Autodesk Inventor part; units mm, degrees
(part 3 of 3)
  line L455 (50.25, -72.75) -> (50.25, -62.25)
  line L456 (50.25, -62.25) -> (24.75, -62.25)
  line L457 (24.75, -62.25) -> (24.75, -72.75)
  line L458 (24.75, -57.75) -> (50.25, -57.75)
  line L459 (50.25, -57.75) -> (50.25, -47.25)
  line L460 (50.25, -47.25) -> (24.75, -47.25)
  line L461 (24.75, -47.25) -> (24.75, -57.75)
  line L462 (24.75, -42.75) -> (50.25, -42.75)
  line L463 (50.25, -42.75) -> (50.25, -32.25)
  line L464 (50.25, -32.25) -> (24.75, -32.25)
  line L465 (24.75, -32.25) -> (24.75, -42.75)
  line L466 (24.75, -27.75) -> (50.25, -27.75)
  line L467 (50.25, -27.75) -> (50.25, -17.25)
  line L468 (50.25, -17.25) -> (24.75, -17.25)
  line L469 (24.75, -17.25) -> (24.75, -27.75)
  line L470 (24.75, -12.75) -> (50.25, -12.75)
  line L471 (50.25, -12.75) -> (50.25, -2.25)
  line L472 (50.25, -2.25) -> (24.75, -2.25)
  line L473 (24.75, -2.25) -> (24.75, -12.75)
  line L474 (24.75, 2.25) -> (50.25, 2.25)
  line L475 (50.25, 2.25) -> (50.25, 12.75)
  line L476 (50.25, 12.75) -> (24.75, 12.75)
  line L477 (24.75, 12.75) -> (24.75, 2.25)
  line L478 (24.75, 17.25) -> (50.25, 17.25)
  line L479 (50.25, 17.25) -> (50.25, 27.75)
  line L480 (50.25, 27.75) -> (24.75, 27.75)
  line L481 (24.75, 27.75) -> (24.75, 17.25)
  line L482 (24.75, 32.25) -> (50.25, 32.25)
  line L483 (50.25, 32.25) -> (50.25, 42.75)
  line L484 (50.25, 42.75) -> (24.75, 42.75)
  line L485 (24.75, 42.75) -> (24.75, 32.25)
  line L486 (24.75, 47.25) -> (50.25, 47.25)
  line L487 (50.25, 47.25) -> (50.25, 57.75)
  line L488 (50.25, 57.75) -> (24.75, 57.75)
  line L489 (24.75, 57.75) -> (24.75, 47.25)
  line L490 (24.75, 62.25) -> (50.25, 62.25)
  line L491 (50.25, 62.25) -> (50.25, 72.75)
  line L492 (50.25, 72.75) -> (24.75, 72.75)
  line L493 (24.75, 72.75) -> (24.75, 62.25)
  line L494 (24.75, 77.25) -> (50.25, 77.25)
  line L495 (50.25, 77.25) -> (50.25, 87.75)
  line L496 (50.25, 87.75) -> (24.75, 87.75)
  line L497 (24.75, 87.75) -> (24.75, 77.25)
  line L498 (24.75, 92.25) -> (50.25, 92.25)
  line L499 (50.25, 92.25) -> (50.25, 102.75)
  line L500 (50.25, 102.75) -> (24.75, 102.75)
  line L501 (24.75, 102.75) -> (24.75, 92.25)
  line L502 (24.75, 107.25) -> (50.25, 107.25)
  line L503 (50.25, 107.25) -> (50.25, 117.75)
  line L504 (50.25, 117.75) -> (24.75, 117.75)
  line L505 (24.75, 117.75) -> (24.75, 107.25)
  line L506 (9.75, -87.75) -> (20.25, -87.75)
  line L507 (20.25, -87.75) -> (20.25, -69.75)
  line L508 (20.25, -69.75) -> (9.75, -69.75)
  line L509 (9.75, -69.75) -> (9.75, -87.75)
  line L510 (9.75, -47.25) -> (20.25, -47.25)
  line L511 (20.25, -47.25) -> (20.25, -65.25)
  line L512 (20.25, -65.25) -> (9.75, -65.25)
  line L513 (9.75, -65.25) -> (9.75, -47.25)
  line L514 (9.75, -42.75) -> (20.25, -42.75)
  line L515 (20.25, -42.75) -> (20.25, -24.75)
  line L516 (20.25, -24.75) -> (9.75, -24.75)
  line L517 (9.75, -24.75) -> (9.75, -42.75)
  line L518 (9.75, -20.25) -> (20.25, -20.25)
  line L519 (20.25, -20.25) -> (20.25, -9.75)
  line L520 (20.25, -9.75) -> (9.75, -9.75)
  line L521 (9.75, -9.75) -> (9.75, -20.25)
  line L522 (9.75, 12.75) -> (20.25, 12.75)
  line L523 (20.25, 12.75) -> (20.25, -5.25)
  line L524 (20.25, -5.25) -> (9.75, -5.25)
  line L525 (9.75, -5.25) -> (9.75, 12.75)
  line L526 (9.75, 17.25) -> (20.25, 17.25)
  line L527 (20.25, 17.25) -> (20.25, 35.25)
  line L528 (20.25, 35.25) -> (9.75, 35.25)
  line L529 (9.75, 35.25) -> (9.75, 17.25)
  line L530 (9.75, 57.75) -> (20.25, 57.75)
  line L531 (20.25, 57.75) -> (20.25, 39.75)
  line L532 (20.25, 39.75) -> (9.75, 39.75)
  line L533 (9.75, 39.75) -> (9.75, 57.75)
  line L534 (9.75, 62.25) -> (20.25, 62.25)
  line L535 (20.25, 62.25) -> (20.25, 80.25)
  line L536 (20.25, 80.25) -> (9.75, 80.25)
  line L537 (9.75, 80.25) -> (9.75, 62.25)
  line L538 (9.75, 117.75) -> (20.25, 117.75)
  line L539 (20.25, 117.75) -> (20.25, 99.75)
  line L540 (20.25, 99.75) -> (9.75, 99.75)
  line L541 (9.75, 99.75) -> (9.75, 117.75)
  line L542 (9.75, 84.75) -> (20.25, 84.75)
  line L543 (20.25, 84.75) -> (20.25, 95.25)
  line L544 (20.25, 95.25) -> (9.75, 95.25)
  line L545 (9.75, 95.25) -> (9.75, 84.75)
  point P0 (0, 0)
  point P1 (9.75, -64.25)
  point P2 (20.25, -53.75)
  point P3 (20.25, -49.25)
  point P4 (20.25, -8.75)
  point P5 (20.25, -4.25)
  point P6 (20.25, 36.25)
  point P7 (9.75, 40.75)
  point P8 (20.25, 51.25)
  point P9 (20.25, 55.75)
  point P10 (20.25, 96.25)
  point P11 (20.25, 100.75)
  point P12 (35.25, 27.75)
  point P13 (39.75, 17.25)
  point P14 (39.75, 27.75)
  point P15 (35.25, 57.75)
  point P16 (35.25, 72.75)
  point P17 (35.25, 77.25)
  point P18 (35.25, 117.75)
  point P19 (35.25, -47.25)
  point P20 (35.25, -77.25)
  point P21 (35.25, -32.25)
  point P22 (39.75, -32.25)
  point P23 (35.25, -17.25)
  point P24 (39.75, -17.25)
  point P25 (39.75, -12.75)
  point P26 (39.75, -2.25)
  point P27 (35.25, 2.25)
  point P28 (39.75, 2.25)
  point P29 (39.75, 12.75)
  point P30 (9.75, 99.75)
  point P31 (20.25, 99.75)
  point P32 (20.25, 102.75)
  point P33 (20.25, 107.25)
  point P34 (9.75, 107.25)
  point P35 (9.75, 102.75)
  point P36 (9.75, 95.25)
  point P37 (9.75, 92.25)
  point P38 (9.75, 87.75)
  point P39 (20.25, 84.75)
  point P40 (20.25, 87.75)
  point P41 (20.25, 92.25)
  point P42 (9.75, 80.25)
  point P43 (9.75, 77.25)
  point P44 (9.75, 72.75)
  point P45 (20.25, 72.75)
  point P46 (9.75, 39.75)
  point P47 (9.75, 47.25)
  point P48 (9.75, 42.75)
  point P49 (20.25, 35.25)
  point P50 (9.75, 35.25)
  point P51 (9.75, 32.25)
  point P52 (9.75, 27.75)
  point P53 (20.25, 27.75)
  point P54 (20.25, 32.25)
  point P55 (9.75, -5.25)
  point P56 (20.25, -5.25)
  point P57 (20.25, -2.25)
  point P58 (20.25, 2.25)
  point P59 (9.75, 2.25)
  point P60 (9.75, -2.25)
  point P61 (9.75, -9.75)
  point P62 (9.75, -12.75)
  point P63 (9.75, -17.25)
  point P64 (20.25, -20.25)
  point P65 (20.25, -17.25)
  point P66 (9.75, -24.75)
  point P67 (9.75, -27.75)
  point P68 (9.75, -32.25)
  point P69 (20.25, -32.25)
  point P70 (9.75, -65.25)
  point P71 (20.25, -62.25)
  point P72 (20.25, -57.75)
  point P73 (9.75, -57.75)
  point P74 (9.75, -62.25)
  point P75 (9.75, -69.75)
  point P76 (9.75, -72.75)
  point P77 (9.75, -77.25)
  point P78 (20.25, -77.25)
  dimension "d223" = 0.25
  dimension "d224" = 10.5
  dimension "d225" = 10.5
  dimension "d226" = 0.25
  dimension "d229" = 15
  dimension "d232" = 15
  dimension "d283" = 10.5
  dimension "d284" = 18
  dimension "d285" = 18
  dimension "d286" = 18
  dimension "d287" = 10.5
  dimension "d288" = 4.5
  dimension "d289" = 18
  dimension "d290" = 18
  dimension "d291" = 18
  dimension "d292" = 18
  dimension "d293" = 18
  dimension "d294" = 10.5
  dimension "d295" = 4.5
  constraints: 1088 end point, 50 parallel, 26 horizontal, 25 perpendicular, 21 point on line, 2 collinear, 1 vertical, 886 other
  measures "d223" distance between parallel lines of L4 L0
  measures "d224" distance of L0.start L0.end
  measures "d225" distance of L0.end L1.end
  measures "d226" distance between parallel lines of L5 L3
  measures "d229" distance of L0.start L6.start
  measures "d232" distance of L0.start L66.start
  measures "d283" distance of L508.end L507.end
  measures "d284" distance of L507.end L506.end
  measures "d285" distance of L510.end L511.end
  measures "d286" distance of L514.end L515.end
  measures "d287" distance of L518.end L519.end
  measures "d288" distance between parallel lines of L516 L518
  measures "d289" distance of L522.end L523.end
  measures "d290" distance of L526.end L527.end
  measures "d291" distance of L530.end L531.end
  measures "d292" distance of L534.end L535.end
  measures "d293" distance of L538.end L539.end
  measures "d294" distance of L542.end L543.end
  measures "d295" distance between parallel lines of L536 L542
extrude "Extrusion8" add sketch "Sketch21" along normal blind 1 contours L0 L1 L2 L3 | L6 L7 L8 L9 | L66 L67 L68 L69 | L70 L71 L72 L73 | L130 L131 L132 L133 | L134 L135 L136 L137 | L162 L163 L164 L165 | L166 L167 L168 L169 | L170 L171 L172 L173 | L174 L175 L176 L177 | L178 L179 L180 L181 | L182 L183 L184 L185 | L186 L187 L188 L189 | L190 L191 L192 L193 | L194 L195 L196 L197 | L198 L199 L200 L201 | L226 L227 L228 L229 | L230 L231 L232 L233 | L234 L235 L236 L237 | L238 L239 L240 L241 | L242 L243 L244 L245 | L246 L247 L248 L249 | L250 L251 L252 L253 | L254 L255 L256 L257 | L258 L259 L260 L261 | L262 L263 L264 L265 | L266 L267 L268 L269 | L268 L509 L270 L507 | L270 L271 L508 L273 | L512 L271 L272 L273 | L272 L513 L274 L511 | L274 L275 L276 L277 | L278 L279 L280 L281 | L280 L517 L282 L515 | L282 L283 L516 L285 | L518 L283 L284 L285 | L284 L521 L286 L519 | L286 L287 L520 L289 | L524 L287 L288 L289 | L288 L525 L290 L523 | L290 L291 L292 L293 | L294 L295 L296 L297 | L296 L529 L298 L527 | L298 L299 L528 L301 | L532 L299 L300 L301 | L300 L533 L302 L531 | L302 L303 L304 L305 | L306 L307 L308 L309 | L308 L537 L310 L535 | L310 L311 L536 L313 | L542 L311 L312 L313 | L312 L545 L314 L543 | L314 L315 L544 L317 | L540 L315 L316 L317 | L316 L541 L318 L539 | L318 L319 L320 L321 | L322 L323 L324 L325 | L326 L327 L328 L329 | L330 L331 L332 L333 | L333 L452 L395 L450 | L395 L396 L397 L394 | L334 L335 L336 L337 | L337 L456 L399 L454 | L399 L400 L401 L398 | L338 L339 L340 L341 | L341 L460 L403 L458 | L403 L404 L405 L402 | L342 L343 L344 L345 | L345 L464 L407 L462 | L407 L408 L409 L406 | L346 L347 L348 L349 | L349 L468 L411 L466 | L411 L412 L413 L410 | L350 L351 L352 L353 | L353 L472 L415 L470 | L415 L416 L417 L414 | L354 L355 L356 L357 | L357 L476 L419 L474 | L419 L420 L421 L418 | L358 L359 L360 L361 | L361 L480 L423 L478 | L423 L424 L425 L422 | L362 L363 L364 L365 | L365 L484 L427 L482 | L427 L428 L429 L426 | L366 L367 L368 L369 | L369 L488 L431 L486 | L431 L432 L433 L430 | L370 L371 L372 L373 | L373 L492 L435 L490 | L435 L436 L437 L434 | L374 L375 L376 L377 | L377 L496 L439 L494 | L439 L440 L441 L438 | L378 L379 L380 L381 | L381 L500 L443 L498 | L443 L444 L445 L442 | L382 L383 L384 L385 | L385 L504 L447 L502 | L447 L448 L449 L446 | L386 L387 L388 L389 | L390 L391 L392 L393
sketch "Sketch23" plane through (0, 4, 0) normal (0, 1, 0) x (1, 0, 0)
  circle A0 centre (-63.5, -131.25) radius 10.25
  line L0 (-60.5, 128.25) -> (-60.5, -128.25) projected
  line L1 (-60.5, -128.25) -> (60.5, -128.25) projected
  circle A1 centre (63.5, 131.25) radius 10.25
  circle A2 centre (63.5, -131.25) radius 10.25
  line L2 (60.5, -128.25) -> (60.5, 128.25) projected
  line L3 (60.5, 128.25) -> (-60.5, 128.25) projected
  circle A3 centre (-63.5, 131.25) radius 10.25
  circle A4 centre (-63.5, 0) radius 5.25
  circle A5 centre (63.5, 0) radius 5.25
  point P0 (0, 0)
  point P1 (-53.6989, -128.25)
  point P2 (-60.5, -121.4489)
  dimension "d338" = 20.5
  dimension "d339" = 3
  dimension "d340" = 3
  dimension "d341" = 20.5
  dimension "d342" = 3
  dimension "d343" = 3
  dimension "d344" = 20.5
  dimension "d345" = 3
  dimension "d346" = 3
  dimension "d347" = 3
  dimension "d348" = 3
  dimension "d349" = 20.5
  dimension "d350" = 10.5
  dimension "d351" = 3
  dimension "d352" = 128.25
  dimension "d353" = 10.5
  dimension "d354" = 3
  dimension "d355" = 128.25
  constraints: 6 centre point
  measures "d338" diameter of A0
  measures "d339" distance from line of L0 A0.centre
  measures "d340" distance from line of A0.centre L1
  measures "d341" diameter of A2
  measures "d342" distance from line of L2 A2.centre
  measures "d343" distance from line of L1 A2.centre
  measures "d344" diameter of A1
  measures "d345" distance from line of L3 A1.centre
  measures "d346" distance from line of L2 A1.centre
  measures "d347" distance from line of L0 A3.centre
  measures "d348" distance from line of L3 A3.centre
  measures "d349" diameter of A3
  measures "d350" diameter of A4
  measures "d351" distance from line of L0 A4.centre
  measures "d352" distance from line of L3 A4.centre
  measures "d353" diameter of A5
  measures "d354" distance from line of L2 A5.centre
  measures "d355" distance from line of L1 A5.centre
extrude "Extrusion9" cut sketch "Sketch23" against normal through all contours L1 L0 A0 | A2 L2 L1 | L1 L2 A2 | A4 L0 | L0 A4 | A5 L2 | L2 A5 | A3 L3 L0 | L0 L3 A3 | L2 L3 A1 | A1 L3 L2 picked at (-59.7398, -124.0546)
sketch "Sketch24" plane through (0, 4, 0) normal (0, 1, 0) x (1, 0, 0)
  line L0 (-52, 0.5) -> (-23, 0.5)
  line L1 (-23, 0.5) -> (-23, 29.5) construction
  line L2 (-23, 29.5) -> (-52, 29.5)
  line L3 (-52, 29.5) -> (-52, 0.5) construction
  line L4 (-52, 30.5) -> (-23, 30.5)
  line L5 (-23, 30.5) -> (-23, 59.5)
  line L6 (-23, 59.5) -> (-52, 59.5)
  line L7 (-52, 59.5) -> (-52, 30.5)
  line L8 (-52, 60.5) -> (-23, 60.5)
  line L9 (-23, 60.5) -> (-23, 89.5)
  line L10 (-23, 89.5) -> (-52, 89.5)
  line L11 (-52, 89.5) -> (-52, 60.5)
  line L12 (-52, 90.5) -> (-23, 90.5)
  line L13 (-23, 90.5) -> (-23, 119.5)
  line L14 (-23, 119.5) -> (-52, 119.5)
  line L15 (-52, 119.5) -> (-52, 90.5)
  line L16 (-60.5, 121.25) -> (-60.5, 4.3084) projected
  line L17 (-52, -0.5) -> (7, -0.5) projected
  line L18 (-43.5, 9) -> (-31.5, 9) construction
  line L19 (-31.5, 9) -> (-31.5, 21) construction
  line L20 (-31.5, 21) -> (-43.5, 21) construction
  line L21 (-43.5, 21) -> (-43.5, 9)
  line L22 (-43.5, 39) -> (-31.5, 39)
  line L23 (-31.5, 39) -> (-31.5, 51)
  line L24 (-31.5, 51) -> (-43.5, 51)
  line L25 (-43.5, 51) -> (-43.5, 39)
  line L26 (-43.5, 69) -> (-31.5, 69)
  line L27 (-31.5, 69) -> (-31.5, 81)
  line L28 (-31.5, 81) -> (-43.5, 81)
  line L29 (-43.5, 81) -> (-43.5, 69)
  line L30 (-43.5, 99) -> (-31.5, 99)
  line L31 (-31.5, 99) -> (-31.5, 111)
  line L32 (-31.5, 111) -> (-43.5, 111)
  line L33 (-43.5, 111) -> (-43.5, 99)
  line L34 (-49.7, 0.1) -> (-43.5, 0.1)
  line L35 (-43.5, 0.1) -> (-43.5, 26.3)
  line L36 (-43.5, 26.3) -> (-49.7, 26.3)
  line L37 (-49.7, 26.3) -> (-49.7, 0.1)
  line L38 (-49.7, 30.1) -> (-43.5, 30.1)
  line L39 (-43.5, 30.1) -> (-43.5, 56.3)
  line L40 (-43.5, 56.3) -> (-49.7, 56.3)
  line L41 (-49.7, 56.3) -> (-49.7, 30.1)
  line L42 (-49.7, 60.1) -> (-43.5, 60.1)
  line L43 (-43.5, 60.1) -> (-43.5, 86.3)
  line L44 (-43.5, 86.3) -> (-49.7, 86.3)
  line L45 (-49.7, 86.3) -> (-49.7, 60.1)
  line L46 (-49.7, 90.1) -> (-43.5, 90.1)
  line L47 (-43.5, 90.1) -> (-43.5, 116.3)
  line L48 (-43.5, 116.3) -> (-49.7, 116.3)
  line L49 (-49.7, 116.3) -> (-49.7, 90.1)
  line L50 (-31.5, 26.3) -> (-27.5, 26.3)
  line L51 (-27.5, 26.3) -> (-27.5, 6.3)
  line L52 (-27.5, 6.3) -> (-31.5, 6.3)
  line L53 (-31.5, 6.3) -> (-31.5, 26.3)
  line L54 (-31.5, 36.3) -> (-27.5, 36.3)
  line L55 (-27.5, 36.3) -> (-27.5, 56.3)
  line L56 (-27.5, 56.3) -> (-31.5, 56.3)
  line L57 (-31.5, 56.3) -> (-31.5, 36.3)
  line L58 (-31.5, 66.3) -> (-27.5, 66.3)
  line L59 (-27.5, 66.3) -> (-27.5, 86.3)
  line L60 (-27.5, 86.3) -> (-31.5, 86.3)
  line L61 (-31.5, 86.3) -> (-31.5, 66.3)
  line L62 (-31.5, 96.3) -> (-27.5, 96.3)
  line L63 (-27.5, 96.3) -> (-27.5, 116.3)
  line L64 (-27.5, 116.3) -> (-31.5, 116.3)
  line L65 (-31.5, 116.3) -> (-31.5, 96.3)
  point P0 (0, 0)
  point P1 (-60.5, 121.4489)
  point P2 (-49.7, 90.5)
  point P3 (-43.5, 90.5)
  point P4 (-43.5, 111)
  point P5 (-49.7, 60.5)
  point P6 (-43.5, 60.5)
  point P7 (-43.5, 69)
  point P8 (-43.5, 81)
  point P9 (-49.7, 30.5)
  point P10 (-43.5, 30.5)
  point P11 (-43.5, 9)
  point P12 (-31.5, 39)
  point P13 (-31.5, 81)
  point P14 (-31.5, 111)
  dimension "d358" = 29
  dimension "d359" = 29
  dimension "d360" = 29
  dimension "d361" = 29
  dimension "d362" = 29
  dimension "d363" = 29
  dimension "d364" = 29
  dimension "d365" = 8.5
  dimension "d366" = 1
  dimension "d367" = 1
  dimension "d368" = 1
  dimension "d369" = 1
  dimension "d370" = 12
  dimension "d371" = 12
  dimension "d372" = 12
  dimension "d373" = 12
  dimension "d374" = 12
  dimension "d375" = 8.5
  dimension "d376" = 8.5
  dimension "d377" = 8.5
  dimension "d378" = 8.5
  dimension "d379" = 8.5
  dimension "d380" = 6.2
  dimension "d381" = 0
  dimension "d382" = 26.2
  dimension "d383" = 5.3
  dimension "d384" = 6.2
  dimension "d385" = 26.2
  dimension "d386" = 5.3
  dimension "d387" = 6.2
  dimension "d388" = 0
  dimension "d389" = 26.2
  dimension "d390" = 5.3
  dimension "d391" = 0
  dimension "d392" = 6.2
  dimension "d393" = 26.2
  dimension "d394" = 5.3
  dimension "d397" = 5.3
  dimension "d398" = 20
  dimension "d399" = 4
  dimension "d400" = 0
  dimension "d401" = 4
  dimension "d402" = 20
  dimension "d403" = 20
  dimension "d404" = 20
  dimension "d405" = 5.3
  dimension "d406" = 5.3
  dimension "d407" = 5.3
  dimension "d408" = 0
  constraints: 128 end point, 32 parallel, 16 horizontal, 16 perpendicular, 15 point on line
  measures "d358" distance of L0.end L1.end
  measures "d359" distance of L1.end L2.end
  measures "d360" distance of L5.end L6.end
  measures "d361" distance of L4.end L5.end
  measures "d362" distance of L8.end L9.end
  measures "d363" distance of L13.end L14.end
  measures "d364" distance of L12.end L13.end
  measures "d365" distance between parallel lines of L16 L3
  measures "d366" distance between parallel lines of L2 L4
  measures "d367" distance between parallel lines of L6 L8
  measures "d368" distance between parallel lines of L10 L12
  measures "d369" distance between parallel lines of L17 L0
  measures "d370" distance of L20.end L18.start
  measures "d371" distance of L19.end L20.end
  measures "d372" distance of L24.end L22.start
  measures "d373" distance of L28.end L26.start
  measures "d374" distance of L32.end L30.start
  measures "d375" distance between parallel lines of L3 L21
  measures "d376" distance between parallel lines of L2 L20
  measures "d377" distance between parallel lines of L4 L22
  measures "d378" distance between parallel lines of L8 L26
  measures "d379" distance between parallel lines of L12 L30
  measures "d380" distance of L35.end L36.end
  measures "d381" distance between parallel lines of L21 L35
  measures "d382" distance of L36.end L34.start
  measures "d383" distance between parallel lines of L20 L36
  measures "d384" distance of L47.end L48.end
  measures "d385" distance of L40.end L38.start
  measures "d386" distance between parallel lines of L40 L24
  measures "d387" distance of L39.end L40.end
  measures "d388" distance between parallel lines of L25 L39
  measures "d389" distance of L42.end L43.end
  measures "d390" distance between parallel lines of L28 L44
  measures "d391" distance between parallel lines of L29 L43
  measures "d392" distance of L43.end L44.end
  measures "d393" distance of L48.end L46.start
  measures "d394" distance between parallel lines of L32 L48
  measures "d397" distance between parallel lines of L20 L50
  measures "d398" distance of L50.end L51.end
  measures "d399" distance of L50.start L50.end
  measures "d400" distance between parallel lines of L19 L53
  measures "d401" distance of L55.end L56.end
  measures "d402" distance of L54.end L55.end
  measures "d403" distance of L58.end L59.end
  measures "d404" distance of L62.end L63.end
  measures "d405" distance between parallel lines of L32 L64
  measures "d406" distance between parallel lines of L28 L60
  measures "d407" distance between parallel lines of L24 L56
  measures "d408" distance between parallel lines of L23 L57
extrude "Extrusion10" add sketch "Sketch24" along normal blind 2.4 contours L37 L36 L35 L21 L0 | L0 L35 L34 L37 | L41 L40 L39 L25 L4 | L23 L57 L56 L55 L54 | L45 L44 L43 L29 L8 | L27 L61 L60 L59 L58 | L49 L48 L47 L33 L12 | L31 L65 L64 L63 L62 | L50 L51 L52 L53
sketch "Sketch25" plane through (0, 6.4, 0) normal (0, 1, 0) x (1, 0, 0)
  circle A0 centre (-46.65, 4.4) radius 1.5 projected
  circle A1 centre (-46.65, 21.1) radius 1.5 projected
  circle A2 centre (-46.65, 34.4) radius 1.5 projected
  circle A3 centre (-46.65, 51.1) radius 1.5 projected
  circle A4 centre (-46.65, 64.4) radius 1.5 projected
  circle A5 centre (-46.65, 81.1) radius 1.5 projected
  circle A6 centre (-46.65, 94.4) radius 1.5 projected
  circle A7 centre (-46.65, 111.1) radius 1.5 projected
  point P0 (0, 0)
  point P1 (-46.65, 34.4)
  point P2 (-46.65, 51.1)
  point P3 (-46.65, 21.1)
  point P4 (-46.65, 4.4)
  point P5 (-46.65, 64.4)
  point P6 (-46.65, 81.1)
  point P7 (-46.65, 94.4)
  point P8 (-46.65, 111.1)
  constraints: 8 coincident
hole "Hole1" at (-46.65, 6.4, -34.4) at (-46.65, 6.4, -51.1) at (-46.65, 6.4, -21.1) at (-46.65, 6.4, -4.4) at (-46.65, 6.4, -64.4) at (-46.65, 6.4, -81.1) at (-46.65, 6.4, -94.4) at (-46.65, 6.4, -111.1) direction (0, -1, 0) diameter 2.2 end through all
body "Solid1"
